Autodesk Fusion 360 part; units mm, degrees
(part 3 of 3)
sketch "Sketch22" plane through (0, 2.3, 0) normal (0, 1, 0) x (-1, 0, 0)
  line L0 (44.9912, 63.1205) -> (40.0888, 52.6073)
  line L1 (40.0888, 52.6073) -> (19.0625, 62.412)
  line L2 (19.0625, 62.412) -> (23.9648, 72.9252)
  line L3 (23.9648, 72.9252) -> (44.9912, 63.1205)
  line L4 (-4.3779, 5.9918) -> (10.4137, 37.7126)
  line L5 (10.4137, 37.7126) -> (26.7273, 30.1055)
  line L6 (26.7273, 30.1055) -> (11.9356, -1.6153)
  line L7 (11.9356, -1.6153) -> (-4.3779, 5.9918)
  line L8 (7.625, -1.9104) -> (19.6238, -16.21)
  line L9 (19.6238, -16.21) -> (18.0917, -17.4956)
  line L10 (18.0917, -17.4956) -> (29.6619, -31.2844)
  line L11 (29.6619, -31.2844) -> (25.0656, -35.1411)
  line L12 (25.0656, -35.1411) -> (41.1353, -54.2922)
  line L13 (41.1353, -54.2922) -> (44.1995, -51.7211)
  line L14 (44.1995, -51.7211) -> (55.7697, -65.5099)
  line L15 (55.7697, -65.5099) -> (64.9622, -57.7964)
  line L16 (64.9622, -57.7964) -> (76.5324, -71.5852)
  line L17 (76.5324, -71.5852) -> (79.5966, -69.0141)
  line L18 (79.5966, -69.0141) -> (91.1667, -82.8029)
  line L19 (91.1667, -82.8029) -> (136.3634, -44.8784)
  line L20 (136.3634, -44.8784) -> (120.2937, -25.7273)
  line L21 (120.2937, -25.7273) -> (117.2295, -28.2985)
  line L22 (117.2295, -28.2985) -> (105.6593, -14.5097)
  line L23 (105.6593, -14.5097) -> (96.4668, -22.2231)
  line L24 (96.4668, -22.2231) -> (84.8966, -8.4343)
  line L25 (84.8966, -8.4343) -> (81.8324, -11.0055)
  line L26 (81.8324, -11.0055) -> (74.7618, -2.579)
  line L27 (74.7618, -2.579) -> (79.358, 1.2777)
  line L28 (79.358, 1.2777) -> (74.8585, 6.6401)
  line L29 (74.8585, 6.6401) -> (92.4775, 21.4242)
  line L30 (92.4775, 21.4242) -> (57.1591, 63.5151)
  line L31 (57.1591, 63.5151) -> (16.4458, 82.5)
  line L32 (16.4458, 82.5) -> (-38.5, 82.5)
  line L33 (-38.5, 82.5) -> (-38.5, 59.5)
  line L34 (-38.5, 59.5) -> (-45.5, 59.5)
  line L35 (-45.5, 59.5) -> (-45.5, 53.5)
  line L36 (-45.5, 53.5) -> (-56.5, 53.5)
  line L37 (-56.5, 53.5) -> (-56.5, 57.5)
  line L38 (-56.5, 57.5) -> (-74.5, 57.5)
  line L39 (-74.5, 57.5) -> (-74.5, 69.5)
  line L40 (-74.5, 69.5) -> (-92.5, 69.5)
  line L41 (-92.5, 69.5) -> (-92.5, 73.5)
  line L42 (-92.5, 73.5) -> (-117.5, 73.5)
  line L43 (-117.5, 73.5) -> (-117.5, 14.5)
  line L44 (-117.5, 14.5) -> (-99.5, 14.5)
  line L45 (-99.5, 14.5) -> (-99.5, 10.5)
  line L46 (-99.5, 10.5) -> (-81.5, 10.5)
  line L47 (-81.5, 10.5) -> (-81.5, -1.5)
  line L48 (-81.5, -1.5) -> (-63.5, -1.5)
  line L49 (-63.5, -1.5) -> (-63.5, -5.5)
  line L50 (-63.5, -5.5) -> (-38.5, -5.5)
  line L51 (-38.5, -5.5) -> (-38.5, 0.5)
  line L52 (-38.5, 0.5) -> (-20.5, 0.5)
  line L53 (-20.5, 0.5) -> (-20.5, 2.5)
  line L54 (-20.5, 2.5) -> (-1.8332, 2.5)
  line L55 (-1.8332, 2.5) -> (-1.3728, 3.4872)
  line L56 (-1.3728, 3.4872) -> (8.0853, -0.9232)
  line L57 (8.0853, -0.9232) -> (7.625, -1.9104)
  line L58 (62.672, 13.3847) -> (72.3139, 1.894)
  line L59 (72.3139, 1.894) -> (60.8232, -7.7478)
  line L60 (60.8232, -7.7478) -> (51.1814, 3.7429)
  line L61 (51.1814, 3.7429) -> (62.672, 13.3847)
  line L62 (92.0203, -32.4812) -> (101.6621, -43.9719)
  line L63 (101.6621, -43.9719) -> (90.1714, -53.6137)
  line L64 (90.1714, -53.6137) -> (80.5296, -42.123)
  line L65 (80.5296, -42.123) -> (92.0203, -32.4812)
  line L66 (49.6493, 2.4573) -> (59.2911, -9.0334)
  line L67 (59.2911, -9.0334) -> (47.8004, -18.6752)
  line L68 (47.8004, -18.6752) -> (38.1586, -7.1845)
  line L69 (38.1586, -7.1845) -> (49.6493, 2.4573)
  line L70 (77.1487, -64.5411) -> (67.5068, -53.0504)
  line L71 (67.5068, -53.0504) -> (78.9975, -43.4086)
  line L72 (78.9975, -43.4086) -> (88.6393, -54.8993)
  line L73 (88.6393, -54.8993) -> (77.1487, -64.5411)
  line L74 (-40.5, 37.5) -> (-25.5, 37.5)
  line L75 (-25.5, 37.5) -> (-25.5, 22.5)
  line L76 (-25.5, 22.5) -> (-40.5, 22.5)
  line L77 (-40.5, 22.5) -> (-40.5, 37.5)
  line L78 (32.1098, -35.7574) -> (43.6004, -26.1156)
  line L79 (43.6004, -26.1156) -> (53.2423, -37.6063)
  line L80 (53.2423, -37.6063) -> (41.7516, -47.2481)
  line L81 (41.7516, -47.2481) -> (32.1098, -35.7574)
  line L82 (69.4087, -47.5383) -> (59.7669, -36.0477)
  line L83 (59.7669, -36.0477) -> (71.2576, -26.4059)
  line L84 (71.2576, -26.4059) -> (80.8994, -37.8965)
  line L85 (80.8994, -37.8965) -> (69.4087, -47.5383)
  line L86 (39.6112, 17.5317) -> (49.253, 6.041)
  line L87 (49.253, 6.041) -> (37.7623, -3.6008)
  line L88 (37.7623, -3.6008) -> (28.1205, 7.8899)
  line L89 (28.1205, 7.8899) -> (39.6112, 17.5317)
  line L90 (-58.5, 33.5) -> (-58.5, 48.5)
  line L91 (-58.5, 48.5) -> (-43.5, 48.5)
  line L92 (-43.5, 48.5) -> (-43.5, 33.5)
  line L93 (-43.5, 33.5) -> (-58.5, 33.5)
  line L94 (119.6774, -32.7715) -> (129.3192, -44.2621)
  line L95 (129.3192, -44.2621) -> (117.8285, -53.904)
  line L96 (117.8285, -53.904) -> (108.1867, -42.4133)
  line L97 (108.1867, -42.4133) -> (119.6774, -32.7715)
  line L98 (-76.5, 18.5) -> (-61.5, 18.5)
  line L99 (-61.5, 18.5) -> (-61.5, 3.5)
  line L100 (-61.5, 3.5) -> (-76.5, 3.5)
  line L101 (-76.5, 3.5) -> (-76.5, 18.5)
  line L102 (73.8632, 35.8293) -> (62.3725, 26.1874)
  line L103 (62.3725, 26.1874) -> (52.7307, 37.6781)
  line L104 (52.7307, 37.6781) -> (64.2214, 47.3199)
  line L105 (64.2214, 47.3199) -> (73.8632, 35.8293)
  line L106 (25.1359, -18.1119) -> (36.6265, -8.4701)
  line L107 (36.6265, -8.4701) -> (46.2683, -19.9607)
  line L108 (46.2683, -19.9607) -> (34.7777, -29.6026)
  line L109 (34.7777, -29.6026) -> (25.1359, -18.1119)
  line L110 (-94.5, 30.5) -> (-79.5, 30.5)
  line L111 (-79.5, 30.5) -> (-79.5, 15.5)
  line L112 (-79.5, 15.5) -> (-94.5, 15.5)
  line L113 (-94.5, 15.5) -> (-94.5, 30.5)
  line L114 (45.1325, -24.83) -> (56.6232, -15.1882)
  line L115 (56.6232, -15.1882) -> (66.265, -26.6789)
  line L116 (66.265, -26.6789) -> (54.7743, -36.3207)
  line L117 (54.7743, -36.3207) -> (45.1325, -24.83)
  line L118 (-112.5, 51.5) -> (-97.5, 51.5)
  line L119 (-97.5, 51.5) -> (-97.5, 36.5)
  line L120 (-97.5, 36.5) -> (-112.5, 36.5)
  line L121 (-112.5, 36.5) -> (-112.5, 51.5)
  line L122 (-22.5, 39.5) -> (-7.5, 39.5)
  line L123 (-7.5, 39.5) -> (-7.5, 24.5)
  line L124 (-7.5, 24.5) -> (-22.5, 24.5)
  line L125 (-22.5, 24.5) -> (-22.5, 39.5)
  line L126 (105.043, -21.5538) -> (114.6848, -33.0445)
  line L127 (114.6848, -33.0445) -> (103.1942, -42.6863)
  line L128 (103.1942, -42.6863) -> (93.5524, -31.1956)
  line L129 (93.5524, -31.1956) -> (105.043, -21.5538)
  line L130 (-15.5, 62.5) -> (-15.5, 77.5)
  line L131 (-15.5, 77.5) -> (-0.5, 77.5)
  line L132 (-0.5, 77.5) -> (-0.5, 62.5)
  line L133 (-0.5, 62.5) -> (-15.5, 62.5)
  line L134 (-40.5, 5.5) -> (-40.5, 20.5)
  line L135 (-40.5, 20.5) -> (-25.5, 20.5)
  line L136 (-25.5, 20.5) -> (-25.5, 5.5)
  line L137 (-25.5, 5.5) -> (-40.5, 5.5)
  line L138 (-58.5, 31.5) -> (-43.5, 31.5)
  line L139 (-43.5, 31.5) -> (-43.5, 16.5)
  line L140 (-43.5, 16.5) -> (-58.5, 16.5)
  line L141 (-58.5, 16.5) -> (-58.5, 31.5)
  line L142 (-22.5, 56.5) -> (-7.5, 56.5)
  line L143 (-7.5, 56.5) -> (-7.5, 41.5)
  line L144 (-7.5, 41.5) -> (-22.5, 41.5)
  line L145 (-22.5, 41.5) -> (-22.5, 56.5)
  line L146 (72.7896, -25.1203) -> (84.2803, -15.4785)
  line L147 (84.2803, -15.4785) -> (93.9221, -26.9691)
  line L148 (93.9221, -26.9691) -> (82.4315, -36.611)
  line L149 (82.4315, -36.611) -> (72.7896, -25.1203)
  line L150 (103.2737, -66.1169) -> (91.783, -75.7587)
  line L151 (91.783, -75.7587) -> (82.1412, -64.2681)
  line L152 (82.1412, -64.2681) -> (93.6319, -54.6263)
  line L153 (93.6319, -54.6263) -> (103.2737, -66.1169)
  line L154 (-33.5, 62.5) -> (-33.5, 77.5)
  line L155 (-33.5, 77.5) -> (-18.5, 77.5)
  line L156 (-18.5, 77.5) -> (-18.5, 62.5)
  line L157 (-18.5, 62.5) -> (-33.5, 62.5)
  line L158 (46.7441, -46.9751) -> (58.2348, -37.3333)
  line L159 (58.2348, -37.3333) -> (67.8766, -48.8239)
  line L160 (67.8766, -48.8239) -> (56.3859, -58.4657)
  line L161 (56.3859, -58.4657) -> (46.7441, -46.9751)
  line L162 (-22.5, 22.5) -> (-7.5, 22.5)
  line L163 (-7.5, 22.5) -> (-7.5, 7.5)
  line L164 (-7.5, 7.5) -> (-22.5, 7.5)
  line L165 (-22.5, 7.5) -> (-22.5, 22.5)
  line L166 (41.1433, 18.8173) -> (52.634, 28.4591)
  line L167 (52.634, 28.4591) -> (62.2758, 16.9684)
  line L168 (62.2758, 16.9684) -> (50.7851, 7.3266)
  line L169 (50.7851, 7.3266) -> (41.1433, 18.8173)
  line L170 (73.9427, 12.3986) -> (64.3009, 23.8893)
  line L171 (64.3009, 23.8893) -> (75.7916, 33.5311)
  line L172 (75.7916, 33.5311) -> (85.4334, 22.0405)
  line L173 (85.4334, 22.0405) -> (73.9427, 12.3986)
  line L174 (-61.5, 52.5) -> (-61.5, 37.5)
  line L175 (-61.5, 37.5) -> (-76.5, 37.5)
  line L176 (-76.5, 37.5) -> (-76.5, 52.5)
  line L177 (-76.5, 52.5) -> (-61.5, 52.5)
  line L178 (-79.5, 49.5) -> (-94.5, 49.5)
  line L179 (-94.5, 49.5) -> (-94.5, 64.5)
  line L180 (-94.5, 64.5) -> (-79.5, 64.5)
  line L181 (-79.5, 64.5) -> (-79.5, 49.5)
  line L182 (-25.5, 54.5) -> (-25.5, 39.5)
  line L183 (-25.5, 39.5) -> (-40.5, 39.5)
  line L184 (-40.5, 39.5) -> (-40.5, 54.5)
  line L185 (-40.5, 54.5) -> (-25.5, 54.5)
  line L186 (-79.5, 47.5) -> (-79.5, 32.5)
  line L187 (-79.5, 32.5) -> (-94.5, 32.5)
  line L188 (-94.5, 32.5) -> (-94.5, 47.5)
  line L189 (-94.5, 47.5) -> (-79.5, 47.5)
  line L190 (-112.5, 19.5) -> (-112.5, 34.5)
  line L191 (-112.5, 34.5) -> (-97.5, 34.5)
  line L192 (-97.5, 34.5) -> (-97.5, 19.5)
  line L193 (-97.5, 19.5) -> (-112.5, 19.5)
  line L194 (36.2303, -4.8864) -> (24.7396, -14.5282)
  line L195 (24.7396, -14.5282) -> (15.0978, -3.0375)
  line L196 (15.0978, -3.0375) -> (26.5884, 6.6043)
  line L197 (26.5884, 6.6043) -> (36.2303, -4.8864)
  line L198 (79.2878, -15.7515) -> (67.7971, -25.3933)
  line L199 (67.7971, -25.3933) -> (58.1553, -13.9026)
  line L200 (58.1553, -13.9026) -> (69.646, -4.2608)
  line L201 (69.646, -4.2608) -> (79.2878, -15.7515)
  line L202 (-58.5, 14.5) -> (-43.5, 14.5)
  line L203 (-43.5, 14.5) -> (-43.5, -0.5)
  line L204 (-43.5, -0.5) -> (-58.5, -0.5)
  line L205 (-58.5, -0.5) -> (-58.5, 14.5)
  line L206 (-76.5, 35.5) -> (-61.5, 35.5)
  line L207 (-61.5, 35.5) -> (-61.5, 20.5)
  line L208 (-61.5, 20.5) -> (-76.5, 20.5)
  line L209 (-76.5, 20.5) -> (-76.5, 35.5)
  line L210 (-112.5, 68.5) -> (-97.5, 68.5)
  line L211 (-97.5, 68.5) -> (-97.5, 53.5)
  line L212 (-97.5, 53.5) -> (-112.5, 53.5)
  line L213 (-112.5, 53.5) -> (-112.5, 68.5)
  line L214 (104.8058, -64.8313) -> (95.164, -53.3407)
  line L215 (95.164, -53.3407) -> (106.6546, -43.6989)
  line L216 (106.6546, -43.6989) -> (116.2964, -55.1895)
  line L217 (116.2964, -55.1895) -> (104.8058, -64.8313)
  line L218 (36.8024, 73.0075) -> (31.3646, 75.5432)
  line L219 (31.3646, 75.5432) -> (29.3783, 71.2836)
  line L220 (29.3783, 71.2836) -> (23.3966, 74.0729)
  line L221 (23.3966, 74.0729) -> (15.9586, 58.1219)
  line L222 (15.9586, 58.1219) -> (21.9402, 55.3326)
  line L223 (21.9402, 55.3326) -> (19.8271, 50.801)
  line L224 (19.8271, 50.801) -> (25.2649, 48.2653)
  line L225 (25.2649, 48.2653) -> (26.4545, 50.8163)
  line L226 (30.7028, 45.7296) -> (25.2649, 48.2653)
  line L227 (32.8159, 50.2612) -> (30.7028, 45.7296)
  line L228 (38.7975, 47.4719) -> (32.8159, 50.2612)
  line L229 (46.2356, 63.4229) -> (38.7975, 47.4719)
  line L230 (40.254, 66.2122) -> (46.2356, 63.4229)
  line L231 (42.2403, 70.4718) -> (40.254, 66.2122)
  line L232 (36.8024, 73.0075) -> (42.2403, 70.4718)
  dimension "d180" = 6
  dimension "d181" = 4.7
  dimension "d182" = 6.6
  dimension "d183" = 17.6
  dimension "d184" = 6.6
  dimension "d185" = 5
  dimension "d186" = 6
  constraint midpoint L31 L218.start
  constraint parallel L31 L218
  constraint perpendicular L3 L219
  constraint perpendicular L219 L220
  constraint perpendicular L31 L221
  constraint perpendicular L221 L222
  constraint perpendicular L222 L223
  constraint perpendicular L223 L224
  constraint perpendicular L224 L225
  constraint symmetric L218.start L225 L232.start
  constraint symmetric L218.end L225 L231.start
  constraint symmetric L219.end L225 L230.start
  constraint symmetric L220.end L225 L229.start
  constraint symmetric L221.end L225 L228.start
  constraint symmetric L222.end L225 L227.start
  constraint symmetric L223.end L225 L226.start
  constraint symmetric L224.end L225 L226.end
  measures "d180" distance of L218.start L218.end
  measures "d181" distance of L218.end L219.end
  measures "d182" distance of L219.end L220.end
  measures "d183" distance of L220.end L221.end
  measures "d184" distance of L221.end L222.end
  measures "d185" distance of L222.end L223.end
  measures "d186" distance of L223.end L224.end
extrude "Extrude22" cut sketch "Sketch22" against normal blind 1.6 contours L31 L218 L219 L220 L221 L222 L223 L224 L226 L227 L228 L229 L230 L231 L232
chamfer "Chamfer4" distance 2 angle 45 2 edges at (-40.254, 1.5, 66.2122) (-29.3783, 1.5, 71.2836)
fillet "Fillet5" radius 5 6 edges at (-78.3806, 3.5, 6.3319) (-139.8854, 3.5, -45.1866) (120, 3.5, 76) (41, 3.5, 62) (41, 3.5, 85) (-95.9996, 3.5, 21.116)
sketch "Sketch23" plane through (0, 7, 0) normal (0, 1, 0) x (-1, 0, 0)
  arc A0 (92.1694, 17.9021) -> (92.7857, 24.9463) centre (88.9554, 21.7323) ccw
  line L0 (92.7857, 24.9463) -> (58.7179, 65.5466)
  line L1 (58.7179, 65.5466) -> (17, 85)
  line L2 (17, 85) -> (-36, 85)
  arc A1 (-36, 85) -> (-41, 80) centre (-36, 80) ccw
  line L3 (-41, 80) -> (-41, 67)
  arc A2 (-46, 62) -> (-41, 67) centre (-46, 67) ccw
  line L4 (-46, 62) -> (-48, 62)
  line L5 (-48, 62) -> (-48, 56)
  line L6 (-48, 56) -> (-54, 56)
  line L7 (-54, 56) -> (-54, 60)
  line L8 (-54, 60) -> (-72, 60)
  line L9 (-72, 60) -> (-72, 72)
  line L10 (-72, 72) -> (-90, 72)
  line L11 (-90, 72) -> (-90, 76)
  line L12 (-90, 76) -> (-115, 76)
  arc A3 (-115, 76) -> (-120, 71) centre (-115, 71) ccw
  line L13 (-120, 71) -> (-120, 12)
  line L14 (-120, 12) -> (-102, 12)
  line L15 (-102, 12) -> (-102, 8)
  line L16 (-102, 8) -> (-84, 8)
  line L17 (-84, 8) -> (-84, -4)
  line L18 (-84, -4) -> (-66, -4)
  line L19 (-66, -4) -> (-66, -8)
  line L20 (-66, -8) -> (-36, -8)
  line L21 (-36, -8) -> (-36, -2)
  line L22 (-36, -2) -> (-18, -2)
  line L23 (-18, -2) -> (-7.0624, -7.1003)
  line L24 (-7.0624, -7.1003) -> (-2.5857, 2.5)
  line L25 (-2.5857, 2.5) -> (-20.5, 2.5)
  line L26 (-20.5, 2.5) -> (-20.5, 0.5)
  line L27 (-20.5, 0.5) -> (-38.5, 0.5)
  line L28 (-38.5, 0.5) -> (-38.5, -5.5)
  line L29 (-38.5, -5.5) -> (-63.5, -5.5)
  line L30 (-63.5, -5.5) -> (-63.5, -1.5)
  line L31 (-63.5, -1.5) -> (-81.5, -1.5)
  line L32 (-81.5, -1.5) -> (-81.5, 10.5)
  line L33 (-81.5, 10.5) -> (-99.5, 10.5)
  line L34 (-99.5, 10.5) -> (-99.5, 14.5)
  line L35 (-99.5, 14.5) -> (-117.5, 14.5)
  line L36 (-117.5, 14.5) -> (-117.5, 73.5)
  line L37 (-117.5, 73.5) -> (-92.5, 73.5)
  line L38 (-92.5, 73.5) -> (-92.5, 69.5)
  line L39 (-92.5, 69.5) -> (-74.5, 69.5)
  line L40 (-74.5, 69.5) -> (-74.5, 57.5)
  line L41 (-74.5, 57.5) -> (-56.5, 57.5)
  line L42 (-56.5, 57.5) -> (-56.5, 53.5)
  line L43 (-56.5, 53.5) -> (-45.5, 53.5)
  line L44 (-45.5, 53.5) -> (-45.5, 59.5)
  line L45 (-45.5, 59.5) -> (-38.5, 59.5)
  line L46 (-38.5, 59.5) -> (-38.5, 82.5)
  line L47 (-38.5, 82.5) -> (16.4458, 82.5)
  line L48 (16.4458, 82.5) -> (57.1591, 63.5151)
  line L49 (57.1591, 63.5151) -> (92.4775, 21.4242)
  line L50 (92.4775, 21.4242) -> (74.8585, 6.6401)
  line L51 (74.8585, 6.6401) -> (79.358, 1.2777)
  line L52 (79.358, 1.2777) -> (74.7618, -2.579)
  line L53 (74.7618, -2.579) -> (81.8324, -11.0055)
  line L54 (81.8324, -11.0055) -> (84.8966, -8.4343)
  line L55 (84.8966, -8.4343) -> (96.4668, -22.2231)
  line L56 (96.4668, -22.2231) -> (105.6593, -14.5097)
  line L57 (105.6593, -14.5097) -> (117.2295, -28.2985)
  line L58 (117.2295, -28.2985) -> (120.2937, -25.7273)
  line L59 (120.2937, -25.7273) -> (136.3634, -44.8784)
  line L60 (136.3634, -44.8784) -> (91.1667, -82.8029)
  line L61 (91.1667, -82.8029) -> (79.5966, -69.0141)
  line L62 (79.5966, -69.0141) -> (76.5324, -71.5852)
  line L63 (76.5324, -71.5852) -> (64.9622, -57.7964)
  line L64 (64.9622, -57.7964) -> (55.7697, -65.5099)
  line L65 (55.7697, -65.5099) -> (44.1995, -51.7211)
  line L66 (44.1995, -51.7211) -> (41.1353, -54.2922)
  line L67 (41.1353, -54.2922) -> (25.0656, -35.1411)
  line L68 (25.0656, -35.1411) -> (29.6619, -31.2844)
  line L69 (29.6619, -31.2844) -> (18.0917, -17.4956)
  line L70 (18.0917, -17.4956) -> (19.6238, -16.21)
  line L71 (19.6238, -16.21) -> (8.1087, -2.4869)
  line L72 (8.1087, -2.4869) -> (3.632, -12.0872)
  line L73 (3.632, -12.0872) -> (14.5696, -17.1875)
  line L74 (14.5696, -17.1875) -> (26.1398, -30.9763)
  line L75 (26.1398, -30.9763) -> (21.5435, -34.833)
  line L76 (21.5435, -34.833) -> (40.8272, -57.8143)
  line L77 (40.8272, -57.8143) -> (43.8913, -55.2432)
  line L78 (43.8913, -55.2432) -> (55.4615, -69.032)
  line L79 (55.4615, -69.032) -> (64.6541, -61.3185)
  line L80 (64.6541, -61.3185) -> (76.2242, -75.1073)
  line L81 (76.2242, -75.1073) -> (79.2884, -72.5362)
  line L82 (79.2884, -72.5362) -> (90.8586, -86.325)
  line L83 (90.8586, -86.325) -> (136.0552, -48.4005)
  arc A4 (136.0552, -48.4005) -> (136.6715, -41.3563) centre (132.8413, -44.5703) ccw
  line L84 (136.6715, -41.3563) -> (120.6018, -22.2052)
  line L85 (120.6018, -22.2052) -> (117.5376, -24.7764)
  line L86 (117.5376, -24.7764) -> (105.9674, -10.9876)
  line L87 (105.9674, -10.9876) -> (96.7749, -18.701)
  line L88 (96.7749, -18.701) -> (85.2047, -4.9122)
  line L89 (85.2047, -4.9122) -> (82.1406, -7.4834)
  line L90 (82.1406, -7.4834) -> (78.2838, -2.8871)
  line L91 (78.2838, -2.8871) -> (82.8801, 0.9696)
  line L92 (82.8801, 0.9696) -> (81.5945, 2.5017)
  arc A5 (82.2108, 9.5459) -> (81.5945, 2.5017) centre (85.4247, 5.7156) ccw
  line L93 (82.2108, 9.5459) -> (92.1694, 17.9021)
  line L94 (15.0562, -14.6559) -> (8.716, -7.1)
  line L95 (8.716, -7.1) -> (6.9543, -10.878)
  line L96 (6.9543, -10.878) -> (15.0562, -14.6559)
  line L97 (-16.3735, 0) -> (-8.2716, -3.778)
  line L98 (-8.2716, -3.778) -> (-6.5099, 0)
  line L99 (-6.5099, 0) -> (-16.3735, 0)
  dimension "d192" = -2.5
extrude "Extrude23" cut sketch "Sketch23" against normal blind 7 contours L94 L95 L96 | L97 L98 L99
fillet "Fillet6" radius 3 4 edges at (-136.3634, 4.65, -44.8784) (-92.4775, 4.65, 21.4242) (38.5, 4.65, 82.5) (117.5, 4.65, 73.5)
fillet "Fillet7" radius 3 2 edges at (-74.8585, 4.65, 6.6401) (38.5, 4.65, 59.5)
extrude "Extrude24" cut 1 faces at (-15.8516, 1.6333, 35.1769) along direction (-0.422618, 0, 0.906308) blind 2
equation "d162 = ( 11.8 / 2 ) * 1 mm"
equation "d163 = ( 11.8 / 2 ) * 1 mm"
equation "d167 = ( 5.7 / 2 ) * 1 mm"
